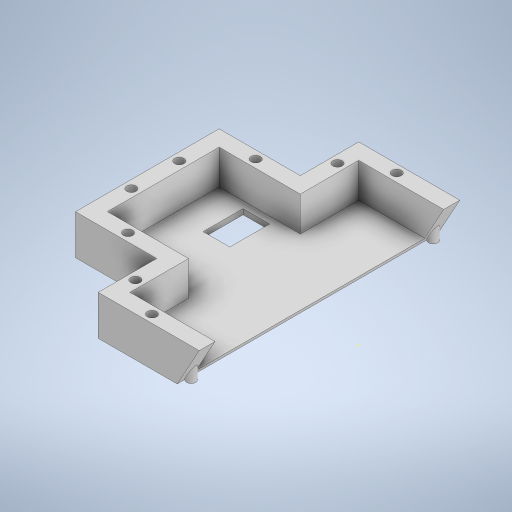
# Autodesk Inventor part: top
Saved by Autodesk Inventor 2023.5 (Build 275446000, 446)
## iProperties
Created: 2025-06-26
Part Number: top
Material: Ogólny
Document SubType Name: Modeling
Designer: karol
Density: 1 g/cm^3
Appearance: Domyślna
Author: karol
Autodesk Inventor part; units mm, degrees
ref_plane "YZ Plane" through (0, 0, 0) normal (1, 0, 0) x (0, 1, 0)
ref_plane "XZ Plane" through (0, 0, 0) normal (0, 1, 0) x (-1, 0, 0)
ref_plane "XY Plane" through (0, 0, 0) normal (0, 0, 1) x (1, 0, 0)
sketch "Szkic1" plane through (0, 0, 0) normal (0, 1, 0) x (-1, 0, 0)
  line L0 (51.2105, 46.6031) -> (4.7105, 46.6031)
  line L1 (4.7105, 46.6031) -> (4.7105, -51.3969)
  line L2 (4.7105, -51.3969) -> (51.2105, -51.3969)
  line L3 (51.2105, -51.3969) -> (51.2105, 46.6031)
  line L4 (51.2105, 46.6031) -> (51.2105, 24.6031)
  line L5 (51.2105, 24.6031) -> (81.7295, 24.6031)
  line L6 (81.7295, 24.6031) -> (81.7295, -29.3969)
  line L7 (81.7295, -29.3969) -> (51.2105, -29.3969)
  line L8 (51.2105, -51.3969) -> (51.2105, -29.3969)
  point P0 (0, 0)
  dimension "d0" = 46.5
  dimension "d1" = 98
  dimension "d2" = 22
  dimension "d3" = 30.519
  dimension "d4" = 54
  constraints: 18 end point, 4 perpendicular, 2 parallel, 2 point on line, 1 collinear, 1 horizontal
  measures "d0" distance of L2.end L1.end
  measures "d1" distance of L1.end L0.end
  measures "d2" distance of L0.start L4.end
  measures "d3" distance of L4.end L5.end
  measures "d4" distance of L5.end L6.end
extrude "Wyciągnięcie proste1" add sketch "Szkic1" along normal blind 15
sketch "Szkic2" plane through (0, 15, 0) normal (0, 1, 0) x (1, 0, 0)
  line L0 (-75.7295, -18.6031) -> (-45.2105, -18.6031)
  line L1 (-45.2105, -18.6031) -> (-45.2105, 23.3969)
  line L2 (-45.2105, 23.3969) -> (-75.7295, 23.3969)
  line L3 (-75.7295, 23.3969) -> (-75.7295, -18.6031)
  line L4 (-81.7295, 29.3969) -> (-81.7295, -24.6031) projected
  line L5 (-81.7295, -24.6031) -> (-51.2105, -24.6031) projected
  line L6 (-45.2105, -40.6509) -> (-10.7105, -40.6509)
  line L7 (-10.7105, -40.6509) -> (-10.7105, 45.3491)
  line L8 (-10.7105, 45.3491) -> (-45.2105, 45.3491)
  line L9 (-45.2105, 45.3491) -> (-45.2105, -40.6509)
  point P0 (0, 0)
  point P1 (-75.7295, 2.3969)
  dimension "d7" = 30.519
  dimension "d8" = 42
  dimension "d9" = 6
  dimension "d10" = 6
  dimension "d11" = 34.5
  dimension "d12" = 86
  constraints: 16 end point, 4 parallel, 2 horizontal, 2 perpendicular, 1 midpoint, 1 point on line
  measures "d7" distance of L2.end L1.end
  measures "d8" distance of L1.end L0.end
  measures "d9" distance from line of L4 point (-75.73, 2.397)
  measures "d10" distance between parallel lines of L5 L0
  measures "d11" distance of L8.end L7.end
  measures "d12" distance of L7.end L6.end
extrude "Wyciągnięcie proste2" cut sketch "Szkic2" against normal blind 13
sketch "Szkic3" plane through (0, 0, 0) normal (0, -1, 0) x (1, 0, 0)
  point P0 (0, 0)
sketch "Szkic4" plane through (0, 0, 0) normal (0, -1, 0) x (1, 0, 0)
  line L0 (-72.6513, -24.862) -> (-72.6513, 21.7196) construction
  line L1 (-72.6513, 21.7196) -> (-57.2809, 21.7196) construction
  line L2 (-57.2809, 21.7196) -> (-57.2809, -24.862) construction
  line L3 (-57.2809, -24.862) -> (-72.6513, -24.862) construction
  line L4 (-66.4228, -19.0142) -> (-66.4228, -19.8248)
  line L5 (-66.4228, -19.8248) -> (-71.6775, -19.8248)
  line L6 (-71.6775, -19.8248) -> (-68.1035, -21.4166)
  line L7 (-68.1035, -21.4166) -> (-68.1035, -21.9109)
  line L8 (-68.1035, -21.9109) -> (-71.6775, -23.4878)
  line L9 (-71.6775, -23.4878) -> (-66.4228, -23.4878)
  line L10 (-66.4228, -23.4878) -> (-66.4228, -24.2441)
  line L11 (-66.4228, -24.2441) -> (-72.5228, -24.2441)
  line L12 (-72.5228, -24.2441) -> (-72.5228, -23.1368)
  line L13 (-72.5228, -23.1368) -> (-69.1267, -21.6143)
  line L14 (-69.1267, -21.6143) -> (-72.5228, -20.1412)
  line L15 (-72.5228, -20.1412) -> (-72.5228, -19.0142)
  line L16 (-72.5228, -19.0142) -> (-66.4228, -19.0142)
  line L17 (-66.4228, -15.6527) -> (-66.4228, -18.0156)
  line L18 (-66.4228, -18.0156) -> (-67.0456, -18.0156)
  line L19 (-67.0456, -18.0156) -> (-67.0456, -17.2395)
  line L20 (-67.0456, -17.2395) -> (-71.8999, -17.2395)
  line L21 (-71.8999, -17.2395) -> (-71.8999, -18.0156)
  line L22 (-71.8999, -18.0156) -> (-72.5228, -18.0156)
  line L23 (-72.5228, -18.0156) -> (-72.5228, -15.6527)
  line L24 (-72.5228, -15.6527) -> (-71.8999, -15.6527)
  line L25 (-71.8999, -15.6527) -> (-71.8999, -16.4288)
  line L26 (-71.8999, -16.4288) -> (-67.0456, -16.4288)
  line L27 (-67.0456, -16.4288) -> (-67.0456, -15.6527)
  line L28 (-67.0456, -15.6527) -> (-66.4228, -15.6527)
  line L29 (-66.4228, -10.2843) -> (-66.4228, -11.1939)
  line L30 (-66.4228, -11.1939) -> (-71.6824, -13.8929)
  line L31 (-71.6824, -13.8929) -> (-66.4228, -13.8929)
  line L32 (-66.4228, -13.8929) -> (-66.4228, -14.6492)
  line L33 (-66.4228, -14.6492) -> (-72.5228, -14.6492)
  line L34 (-72.5228, -14.6492) -> (-72.5228, -13.4975)
  line L35 (-72.5228, -13.4975) -> (-67.6932, -11.0407)
  line L36 (-67.6932, -11.0407) -> (-72.5228, -11.0407)
  line L37 (-72.5228, -11.0407) -> (-72.5228, -10.2843)
  line L38 (-72.5228, -10.2843) -> (-66.4228, -10.2843)
  line L39 (-66.4228, -6.9229) -> (-66.4228, -9.2858)
  line L40 (-66.4228, -9.2858) -> (-67.0456, -9.2858)
  line L41 (-67.0456, -9.2858) -> (-67.0456, -8.5097)
  line L42 (-67.0456, -8.5097) -> (-71.8999, -8.5097)
  line L43 (-71.8999, -8.5097) -> (-71.8999, -9.2858)
  line L44 (-71.8999, -9.2858) -> (-72.5228, -9.2858)
  line L45 (-72.5228, -9.2858) -> (-72.5228, -6.9229)
  line L46 (-72.5228, -6.9229) -> (-71.8999, -6.9229)
  line L47 (-71.8999, -6.9229) -> (-71.8999, -7.699)
  line L48 (-71.8999, -7.699) -> (-67.0456, -7.699)
  line L49 (-67.0456, -7.699) -> (-67.0456, -6.9229)
  line L50 (-67.0456, -6.9229) -> (-66.4228, -6.9229)
  spline S0 degree 2 poles (-68.2963, -1.7819) (-67.8415, -1.7819) (-67.1445, -2.1279) (-66.9171, -2.4146) knots 0 0 0 1 2 2 2
  spline S1 degree 2 poles (-66.9171, -2.4146) (-66.6502, -2.7607) (-66.4228, -3.5466) (-66.4228, -4.1695) knots 0 0 0 1 2 2 2
  line L51 (-66.4228, -4.1695) -> (-66.4228, -5.9194)
  line L52 (-66.4228, -5.9194) -> (-72.5228, -5.9194)
  line L53 (-72.5228, -5.9194) -> (-72.5228, -4.303)
  spline S2 degree 2 poles (-72.5228, -4.303) (-72.5228, -3.6505) (-72.4387, -2.9979) (-72.2756, -2.7013) knots 0 0 0 1 2 2 2
  spline S3 degree 2 poles (-72.2756, -2.7013) (-72.1026, -2.3701) (-71.5341, -2.0686) (-71.1485, -2.0686) knots 0 0 0 1 2 2 2
  spline S4 degree 2 poles (-71.1485, -2.0686) (-70.7185, -2.0686) (-70.0363, -2.5234) (-69.8435, -2.9238) knots 0 0 0 1 2 2 2
  line L54 (-69.8435, -2.9238) -> (-69.8139, -2.9238)
  spline S5 degree 2 poles (-69.8139, -2.9238) (-69.6656, -2.38) (-68.8796, -1.7819) (-68.2963, -1.7819) knots 0 0 0 1 2 2 2
  spline S6 degree 2 poles (-68.2617, -2.6272) (-68.6077, -2.6272) (-69.0526, -2.8249) (-69.2108, -3.1215) knots 0 0 0 1 2 2 2
  spline S7 degree 2 poles (-69.2108, -3.1215) (-69.3096, -3.3143) (-69.369, -3.7691) (-69.369, -4.1893) knots 0 0 0 1 2 2 2
  line L55 (-69.369, -4.1893) -> (-69.369, -5.1087)
  line L56 (-69.369, -5.1087) -> (-67.1148, -5.1087)
  line L57 (-67.1148, -5.1087) -> (-67.1148, -4.4513)
  spline S8 degree 2 poles (-67.1148, -4.4513) (-67.1148, -3.9174) (-67.2137, -3.3044) (-67.3719, -3.0672) knots 0 0 0 1 2 2 2
  spline S9 degree 2 poles (-67.3719, -3.0672) (-67.535, -2.8398) (-67.9403, -2.6272) (-68.2617, -2.6272) knots 0 0 0 1 2 2 2
  spline S10 degree 2 poles (-71.0348, -2.9139) (-71.2523, -2.9139) (-71.5786, -3.0622) (-71.6725, -3.2253) knots 0 0 0 1 2 2 2
  spline S11 degree 2 poles (-71.6725, -3.2253) (-71.7813, -3.4231) (-71.8307, -3.9026) (-71.8307, -4.3326) knots 0 0 0 1 2 2 2
  line L58 (-71.8307, -4.3326) -> (-71.8307, -5.1087)
  line L59 (-71.8307, -5.1087) -> (-70.0462, -5.1087)
  line L60 (-70.0462, -5.1087) -> (-70.0462, -4.1893)
  spline S12 degree 2 poles (-70.0462, -4.1893) (-70.0462, -3.8086) (-70.1253, -3.4478) (-70.2489, -3.255) knots 0 0 0 1 2 2 2
  spline S13 degree 2 poles (-70.2489, -3.255) (-70.3675, -3.0672) (-70.7481, -2.9139) (-71.0348, -2.9139) knots 0 0 0 1 2 2 2
  spline S14 degree 2 poles (-71.8258, 3.3393) (-71.4204, 3.6854) (-70.234, 4.0709) (-69.4728, 4.0709) knots 0 0 0 1 2 2 2
  spline S15 degree 2 poles (-69.4728, 4.0709) (-68.7313, 4.0709) (-67.5301, 3.6952) (-67.1247, 3.3393) knots 0 0 0 1 2 2 2
  spline S16 degree 2 poles (-67.1247, 3.3393) (-66.6996, 2.9636) (-66.2942, 1.97) (-66.2942, 1.3719) knots 0 0 0 1 2 2 2
  spline S17 degree 2 poles (-66.2942, 1.3719) (-66.2942, 0.754) (-66.7144, -0.2347) (-67.1247, -0.5955) knots 0 0 0 1 2 2 2
  spline S18 degree 2 poles (-67.1247, -0.5955) (-67.5301, -0.9465) (-68.7214, -1.3222) (-69.4728, -1.3222) knots 0 0 0 1 2 2 2
  spline S19 degree 2 poles (-69.4728, -1.3222) (-70.239, -1.3222) (-71.4056, -0.9415) (-71.8258, -0.5906) knots 0 0 0 1 2 2 2
  spline S20 degree 2 poles (-71.8258, -0.5906) (-72.2311, -0.2347) (-72.6513, 0.7589) (-72.6513, 1.3719) knots 0 0 0 1 2 2 2
  spline S21 degree 2 poles (-72.6513, 1.3719) (-72.6513, 1.9948) (-72.2163, 2.9933) (-71.8258, 3.3393) knots 0 0 0 1 2 2 2
  spline S22 degree 2 poles (-69.4728, 3.2256) (-70.0758, 3.2256) (-71.0101, 2.9636) (-71.3166, 2.7264) knots 0 0 0 1 2 2 2
  spline S23 degree 2 poles (-71.3166, 2.7264) (-71.633, 2.4841) (-71.9493, 1.802) (-71.9493, 1.3769) knots 0 0 0 1 2 2 2
  spline S24 degree 2 poles (-71.9493, 1.3769) (-71.9493, 0.9369) (-71.6429, 0.2745) (-71.3166, 0.0224) knots 0 0 0 1 2 2 2
  spline S25 degree 2 poles (-71.3166, 0.0224) (-71.0052, -0.2198) (-70.066, -0.4769) (-69.4728, -0.4769) knots 0 0 0 1 2 2 2
  spline S26 degree 2 poles (-69.4728, -0.4769) (-68.2715, -0.4769) (-66.9962, 0.5316) (-66.9962, 1.3769) knots 0 0 0 1 2 2 2
  spline S27 degree 2 poles (-66.9962, 1.3769) (-66.9962, 2.2222) (-68.2715, 3.2256) (-69.4728, 3.2256) knots 0 0 0 1 2 2 2
  line L61 (-66.4228, 8.4952) -> (-66.4228, 4.9607)
  line L62 (-66.4228, 4.9607) -> (-72.5228, 4.9607)
  line L63 (-72.5228, 4.9607) -> (-72.5228, 5.7714)
  line L64 (-72.5228, 5.7714) -> (-67.1445, 5.7714)
  line L65 (-67.1445, 5.7714) -> (-67.1445, 8.4952)
  line L66 (-67.1445, 8.4952) -> (-66.4228, 8.4952)
  line L67 (-66.4228, 10.5565) -> (-71.801, 10.5565)
  line L68 (-71.801, 10.5565) -> (-71.801, 8.51)
  line L69 (-71.801, 8.51) -> (-72.5228, 8.51)
  line L70 (-72.5228, 8.51) -> (-72.5228, 13.4137)
  line L71 (-72.5228, 13.4137) -> (-71.801, 13.4137)
  line L72 (-71.801, 13.4137) -> (-71.801, 11.3672)
  line L73 (-71.801, 11.3672) -> (-66.4228, 11.3672)
  line L74 (-66.4228, 11.3672) -> (-66.4228, 10.5565)
  line L75 (-60.0728, 0.0946) -> (-60.0728, -0.8738)
  line L76 (-60.0728, -0.8738) -> (-61.2365, -1.755)
  line L77 (-61.2365, -1.755) -> (-61.2365, -2.0427)
  line L78 (-61.2365, -2.0427) -> (-60.0728, -2.0427)
  line L79 (-60.0728, -2.0427) -> (-60.0728, -2.8339)
  line L80 (-60.0728, -2.8339) -> (-63.2428, -2.8339)
  line L81 (-63.2428, -2.8339) -> (-63.2428, -1.5597)
  spline S28 degree 2 poles (-63.2428, -1.5597) (-63.2428, -1.2951) (-63.176, -0.9047) (-63.0732, -0.7377) knots 0 0 0 1 2 2 2
  spline S29 degree 2 poles (-63.0732, -0.7377) (-62.9653, -0.5681) (-62.6288, -0.3678) (-62.3719, -0.3678) knots 0 0 0 1 2 2 2
  spline S30 degree 2 poles (-62.3719, -0.3678) (-62.0097, -0.3678) (-61.555, -0.6966) (-61.4214, -0.9714) knots 0 0 0 1 2 2 2
  line L82 (-61.4214, -0.9714) -> (-60.0728, 0.0946)
  spline S31 degree 2 poles (-62.2717, -1.1847) (-62.3925, -1.1847) (-62.5646, -1.2771) (-62.6108, -1.3825) knots 0 0 0 1 2 2 2
  spline S32 degree 2 poles (-62.6108, -1.3825) (-62.6417, -1.457) (-62.6596, -1.6394) (-62.6596, -1.7755) knots 0 0 0 1 2 2 2
  line L83 (-62.6596, -1.7755) -> (-62.6596, -2.0427)
  line L84 (-62.6596, -2.0427) -> (-61.8068, -2.0427)
  line L85 (-61.8068, -2.0427) -> (-61.8068, -1.814)
  spline S33 degree 2 poles (-61.8068, -1.814) (-61.8068, -1.6496) (-61.8479, -1.4159) (-61.9121, -1.3362) knots 0 0 0 1 2 2 2
  spline S34 degree 2 poles (-61.9121, -1.3362) (-61.9737, -1.2592) (-62.1382, -1.1847) (-62.2717, -1.1847) knots 0 0 0 1 2 2 2
  spline S35 degree 2 poles (-61.6578, 3.2158) (-60.8871, 3.2158) (-60.006, 2.3938) (-60.006, 1.6796) knots 0 0 0 1 2 2 2
  spline S36 degree 2 poles (-60.006, 1.6796) (-60.006, 0.9629) (-60.8974, 0.146) (-61.6578, 0.146) knots 0 0 0 1 2 2 2
  spline S37 degree 2 poles (-61.6578, 0.146) (-62.4207, 0.146) (-63.3096, 0.9629) (-63.3096, 1.6796) knots 0 0 0 1 2 2 2
  spline S38 degree 2 poles (-63.3096, 1.6796) (-63.3096, 2.3938) (-62.4259, 3.2158) (-61.6578, 3.2158) knots 0 0 0 1 2 2 2
  spline S39 degree 2 poles (-61.6578, 2.3938) (-61.9429, 2.3938) (-62.3411, 2.2782) (-62.467, 2.178) knots 0 0 0 1 2 2 2
  spline S40 degree 2 poles (-62.467, 2.178) (-62.598, 2.0778) (-62.711, 1.8209) (-62.711, 1.6822) knots 0 0 0 1 2 2 2
  spline S41 degree 2 poles (-62.711, 1.6822) (-62.711, 1.5358) (-62.6057, 1.2969) (-62.4721, 1.1864) knots 0 0 0 1 2 2 2
  spline S42 degree 2 poles (-62.4721, 1.1864) (-62.3488, 1.0888) (-61.9403, 0.9681) (-61.6578, 0.9681) knots 0 0 0 1 2 2 2
  spline S43 degree 2 poles (-61.6578, 0.9681) (-61.3649, 0.9681) (-60.9796, 1.0837) (-60.8486, 1.1838) knots 0 0 0 1 2 2 2
  spline S44 degree 2 poles (-60.8486, 1.1838) (-60.7176, 1.284) (-60.6045, 1.5435) (-60.6045, 1.6822) knots 0 0 0 1 2 2 2
  spline S45 degree 2 poles (-60.6045, 1.6822) (-60.6045, 1.8235) (-60.7253, 2.0855) (-60.8537, 2.1806) knots 0 0 0 1 2 2 2
  spline S46 degree 2 poles (-60.8537, 2.1806) (-60.9924, 2.2833) (-61.3598, 2.3938) (-61.6578, 2.3938) knots 0 0 0 1 2 2 2
  spline S47 degree 2 poles (-61.0438, 6.2214) (-60.8075, 6.2214) (-60.4504, 6.0416) (-60.3322, 5.8926) knots 0 0 0 1 2 2 2
  spline S48 degree 2 poles (-60.3322, 5.8926) (-60.1909, 5.7128) (-60.0728, 5.2863) (-60.0728, 4.955) knots 0 0 0 1 2 2 2
  line L86 (-60.0728, 4.955) -> (-60.0728, 3.6885)
  line L87 (-60.0728, 3.6885) -> (-63.2428, 3.6885)
  line L88 (-63.2428, 3.6885) -> (-63.2428, 4.806)
  spline S49 degree 2 poles (-63.2428, 4.806) (-63.2428, 5.1553) (-63.1888, 5.515) (-63.1041, 5.6717) knots 0 0 0 1 2 2 2
  spline S50 degree 2 poles (-63.1041, 5.6717) (-63.0141, 5.8438) (-62.7059, 6.0108) (-62.5055, 6.0108) knots 0 0 0 1 2 2 2
  spline S51 degree 2 poles (-62.5055, 6.0108) (-62.2743, 6.0108) (-61.9121, 5.7796) (-61.8273, 5.5741) knots 0 0 0 1 2 2 2
  line L89 (-61.8273, 5.5741) -> (-61.8119, 5.5741)
  spline S52 degree 2 poles (-61.8119, 5.5741) (-61.7503, 5.8695) (-61.3675, 6.2214) (-61.0438, 6.2214) knots 0 0 0 1 2 2 2
  spline S53 degree 2 poles (-61.0567, 5.3994) (-61.2056, 5.3994) (-61.3726, 5.2812) (-61.4163, 5.163) knots 0 0 0 1 2 2 2
  spline S54 degree 2 poles (-61.4163, 5.163) (-61.4446, 5.0911) (-61.4497, 4.8368) (-61.4497, 4.6261) knots 0 0 0 1 2 2 2
  line L90 (-61.4497, 4.6261) -> (-61.4497, 4.4797)
  line L91 (-61.4497, 4.4797) -> (-60.6508, 4.4797)
  line L92 (-60.6508, 4.4797) -> (-60.6508, 4.5234)
  spline S55 degree 2 poles (-60.6508, 4.5234) (-60.6508, 4.8317) (-60.6585, 5.068) (-60.7124, 5.1913) knots 0 0 0 1 2 2 2
  spline S56 degree 2 poles (-60.7124, 5.1913) (-60.7612, 5.2992) (-60.9411, 5.3994) (-61.0567, 5.3994) knots 0 0 0 1 2 2 2
  spline S57 degree 2 poles (-62.3488, 5.2016) (-62.4259, 5.2016) (-62.5877, 5.1219) (-62.6237, 5.0397) knots 0 0 0 1 2 2 2
  spline S58 degree 2 poles (-62.6237, 5.0397) (-62.6596, 4.9627) (-62.6648, 4.7469) (-62.6648, 4.5337) knots 0 0 0 1 2 2 2
  line L93 (-62.6648, 4.5337) -> (-62.6648, 4.4797)
  line L94 (-62.6648, 4.4797) -> (-61.9917, 4.4797)
  line L95 (-61.9917, 4.4797) -> (-61.9917, 4.5799)
  spline S59 degree 2 poles (-61.9917, 4.5799) (-61.9917, 4.7828) (-61.9994, 4.9473) (-62.0405, 5.0346) knots 0 0 0 1 2 2 2
  spline S60 degree 2 poles (-62.0405, 5.0346) (-62.0868, 5.1296) (-62.2435, 5.2016) (-62.3488, 5.2016) knots 0 0 0 1 2 2 2
  spline S61 degree 2 poles (-61.6578, 9.5635) (-60.8871, 9.5635) (-60.006, 8.7415) (-60.006, 8.0273) knots 0 0 0 1 2 2 2
  spline S62 degree 2 poles (-60.006, 8.0273) (-60.006, 7.3106) (-60.8974, 6.4937) (-61.6578, 6.4937) knots 0 0 0 1 2 2 2
  spline S63 degree 2 poles (-61.6578, 6.4937) (-62.4207, 6.4937) (-63.3096, 7.3106) (-63.3096, 8.0273) knots 0 0 0 1 2 2 2
  spline S64 degree 2 poles (-63.3096, 8.0273) (-63.3096, 8.7415) (-62.4259, 9.5635) (-61.6578, 9.5635) knots 0 0 0 1 2 2 2
  spline S65 degree 2 poles (-61.6578, 8.7415) (-61.9429, 8.7415) (-62.3411, 8.6259) (-62.467, 8.5257) knots 0 0 0 1 2 2 2
  spline S66 degree 2 poles (-62.467, 8.5257) (-62.598, 8.4255) (-62.711, 8.1686) (-62.711, 8.0299) knots 0 0 0 1 2 2 2
  spline S67 degree 2 poles (-62.711, 8.0299) (-62.711, 7.8835) (-62.6057, 7.6446) (-62.4721, 7.5341) knots 0 0 0 1 2 2 2
  spline S68 degree 2 poles (-62.4721, 7.5341) (-62.3488, 7.4365) (-61.9403, 7.3158) (-61.6578, 7.3158) knots 0 0 0 1 2 2 2
  spline S69 degree 2 poles (-61.6578, 7.3158) (-61.3649, 7.3158) (-60.9796, 7.4314) (-60.8486, 7.5316) knots 0 0 0 1 2 2 2
  spline S70 degree 2 poles (-60.8486, 7.5316) (-60.7176, 7.6317) (-60.6045, 7.8912) (-60.6045, 8.0299) knots 0 0 0 1 2 2 2
  spline S71 degree 2 poles (-60.6045, 8.0299) (-60.6045, 8.1712) (-60.7253, 8.4332) (-60.8537, 8.5283) knots 0 0 0 1 2 2 2
  spline S72 degree 2 poles (-60.8537, 8.5283) (-60.9924, 8.631) (-61.3598, 8.7415) (-61.6578, 8.7415) knots 0 0 0 1 2 2 2
  line L96 (-60.0728, 11.6135) -> (-60.0728, 9.9078)
  line L97 (-60.0728, 9.9078) -> (-60.6251, 9.9078)
  line L98 (-60.6251, 9.9078) -> (-60.6251, 10.3625)
  line L99 (-60.6251, 10.3625) -> (-62.6905, 10.3625)
  line L100 (-62.6905, 10.3625) -> (-62.6905, 9.9078)
  line L101 (-62.6905, 9.9078) -> (-63.2428, 9.9078)
  line L102 (-63.2428, 9.9078) -> (-63.2428, 11.6135)
  line L103 (-63.2428, 11.6135) -> (-62.6905, 11.6135)
  line L104 (-62.6905, 11.6135) -> (-62.6905, 11.1588)
  line L105 (-62.6905, 11.1588) -> (-60.6251, 11.1588)
  line L106 (-60.6251, 11.1588) -> (-60.6251, 11.6135)
  line L107 (-60.6251, 11.6135) -> (-60.0728, 11.6135)
  line L108 (-60.0728, 14.2569) -> (-60.0728, 12.1427)
  line L109 (-60.0728, 12.1427) -> (-63.2428, 12.1427)
  line L110 (-63.2428, 12.1427) -> (-63.2428, 12.939)
  line L111 (-63.2428, 12.939) -> (-60.6765, 12.939)
  line L112 (-60.6765, 12.939) -> (-60.6765, 14.2569)
  line L113 (-60.6765, 14.2569) -> (-60.0728, 14.2569)
  spline S73 degree 2 poles (-61.6578, 17.5219) (-60.8871, 17.5219) (-60.006, 16.6999) (-60.006, 15.9857) knots 0 0 0 1 2 2 2
  spline S74 degree 2 poles (-60.006, 15.9857) (-60.006, 15.269) (-60.8974, 14.4521) (-61.6578, 14.4521) knots 0 0 0 1 2 2 2
  spline S75 degree 2 poles (-61.6578, 14.4521) (-62.4207, 14.4521) (-63.3096, 15.269) (-63.3096, 15.9857) knots 0 0 0 1 2 2 2
  spline S76 degree 2 poles (-63.3096, 15.9857) (-63.3096, 16.6999) (-62.4259, 17.5219) (-61.6578, 17.5219) knots 0 0 0 1 2 2 2
  spline S77 degree 2 poles (-61.6578, 16.6999) (-61.9429, 16.6999) (-62.3411, 16.5843) (-62.467, 16.4841) knots 0 0 0 1 2 2 2
  spline S78 degree 2 poles (-62.467, 16.4841) (-62.598, 16.3839) (-62.711, 16.127) (-62.711, 15.9883) knots 0 0 0 1 2 2 2
  spline S79 degree 2 poles (-62.711, 15.9883) (-62.711, 15.8419) (-62.6057, 15.603) (-62.4721, 15.4925) knots 0 0 0 1 2 2 2
  spline S80 degree 2 poles (-62.4721, 15.4925) (-62.3488, 15.3949) (-61.9403, 15.2742) (-61.6578, 15.2742) knots 0 0 0 1 2 2 2
  spline S81 degree 2 poles (-61.6578, 15.2742) (-61.3649, 15.2742) (-60.9796, 15.3898) (-60.8486, 15.4899) knots 0 0 0 1 2 2 2
  spline S82 degree 2 poles (-60.8486, 15.4899) (-60.7176, 15.5901) (-60.6045, 15.8496) (-60.6045, 15.9883) knots 0 0 0 1 2 2 2
  spline S83 degree 2 poles (-60.6045, 15.9883) (-60.6045, 16.1296) (-60.7253, 16.3916) (-60.8537, 16.4867) knots 0 0 0 1 2 2 2
  spline S84 degree 2 poles (-60.8537, 16.4867) (-60.9924, 16.5894) (-61.3598, 16.6999) (-61.6578, 16.6999) knots 0 0 0 1 2 2 2
  point P0 (0, 0)
  constraints: 2 other
extrude "Wyciągnięcie proste3" add sketch "Szkic4" against normal blind 1
sketch "Szkic5" plane through (0, 0, 0) normal (0, -1, 0) x (1, 0, 0)
  point P0 (0, 0)
sketch "Szkic6" plane through (0, 0, 0) normal (0, -1, 0) x (1, 0, 0)
  line L0 (-74.9036, -23.2743) -> (-74.9036, 27.821) construction
  line L1 (-74.9036, 27.821) -> (-59.7073, 27.821) construction
  line L2 (-59.7073, 27.821) -> (-59.7073, -23.2743) construction
  line L3 (-59.7073, -23.2743) -> (-74.9036, -23.2743) construction
  line L4 (-68.6751, -17.4264) -> (-68.6751, -18.2371)
  line L5 (-68.6751, -18.2371) -> (-73.9298, -18.2371)
  line L6 (-73.9298, -18.2371) -> (-70.3558, -19.8289)
  line L7 (-70.3558, -19.8289) -> (-70.3558, -20.3232)
  line L8 (-70.3558, -20.3232) -> (-73.9298, -21.9001)
  line L9 (-73.9298, -21.9001) -> (-68.6751, -21.9001)
  line L10 (-68.6751, -21.9001) -> (-68.6751, -22.6564)
  line L11 (-68.6751, -22.6564) -> (-74.7751, -22.6564)
  line L12 (-74.7751, -22.6564) -> (-74.7751, -21.5491)
  line L13 (-74.7751, -21.5491) -> (-71.379, -20.0266)
  line L14 (-71.379, -20.0266) -> (-74.7751, -18.5535)
  line L15 (-74.7751, -18.5535) -> (-74.7751, -17.4264)
  line L16 (-74.7751, -17.4264) -> (-68.6751, -17.4264)
  line L17 (-68.6751, -14.065) -> (-68.6751, -16.4279)
  line L18 (-68.6751, -16.4279) -> (-69.2979, -16.4279)
  line L19 (-69.2979, -16.4279) -> (-69.2979, -15.6518)
  line L20 (-69.2979, -15.6518) -> (-74.1522, -15.6518)
  line L21 (-74.1522, -15.6518) -> (-74.1522, -16.4279)
  line L22 (-74.1522, -16.4279) -> (-74.7751, -16.4279)
  line L23 (-74.7751, -16.4279) -> (-74.7751, -14.065)
  line L24 (-74.7751, -14.065) -> (-74.1522, -14.065)
  line L25 (-74.1522, -14.065) -> (-74.1522, -14.8411)
  line L26 (-74.1522, -14.8411) -> (-69.2979, -14.8411)
  line L27 (-69.2979, -14.8411) -> (-69.2979, -14.065)
  line L28 (-69.2979, -14.065) -> (-68.6751, -14.065)
  line L29 (-68.6751, -8.6966) -> (-68.6751, -9.6062)
  line L30 (-68.6751, -9.6062) -> (-73.9347, -12.3052)
  line L31 (-73.9347, -12.3052) -> (-68.6751, -12.3052)
  line L32 (-68.6751, -12.3052) -> (-68.6751, -13.0615)
  line L33 (-68.6751, -13.0615) -> (-74.7751, -13.0615)
  line L34 (-74.7751, -13.0615) -> (-74.7751, -11.9097)
  line L35 (-74.7751, -11.9097) -> (-69.9455, -9.4529)
  line L36 (-69.9455, -9.4529) -> (-74.7751, -9.4529)
  line L37 (-74.7751, -9.4529) -> (-74.7751, -8.6966)
  line L38 (-74.7751, -8.6966) -> (-68.6751, -8.6966)
  line L39 (-68.6751, -5.3352) -> (-68.6751, -7.6981)
  line L40 (-68.6751, -7.6981) -> (-69.2979, -7.6981)
  line L41 (-69.2979, -7.6981) -> (-69.2979, -6.922)
  line L42 (-69.2979, -6.922) -> (-74.1522, -6.922)
  line L43 (-74.1522, -6.922) -> (-74.1522, -7.6981)
  line L44 (-74.1522, -7.6981) -> (-74.7751, -7.6981)
  line L45 (-74.7751, -7.6981) -> (-74.7751, -5.3352)
  line L46 (-74.7751, -5.3352) -> (-74.1522, -5.3352)
  line L47 (-74.1522, -5.3352) -> (-74.1522, -6.1113)
  line L48 (-74.1522, -6.1113) -> (-69.2979, -6.1113)
  line L49 (-69.2979, -6.1113) -> (-69.2979, -5.3352)
  line L50 (-69.2979, -5.3352) -> (-68.6751, -5.3352)
  spline S0 degree 2 poles (-70.5486, -0.1942) (-70.0938, -0.1942) (-69.3968, -0.5402) (-69.1694, -0.8269) knots 0 0 0 1 2 2 2
  spline S1 degree 2 poles (-69.1694, -0.8269) (-68.9025, -1.1729) (-68.6751, -1.9589) (-68.6751, -2.5818) knots 0 0 0 1 2 2 2
  line L51 (-68.6751, -2.5818) -> (-68.6751, -4.3317)
  line L52 (-68.6751, -4.3317) -> (-74.7751, -4.3317)
  line L53 (-74.7751, -4.3317) -> (-74.7751, -2.7152)
  spline S2 degree 2 poles (-74.7751, -2.7152) (-74.7751, -2.0627) (-74.691, -1.4102) (-74.5279, -1.1136) knots 0 0 0 1 2 2 2
  spline S3 degree 2 poles (-74.5279, -1.1136) (-74.3549, -0.7824) (-73.7864, -0.4809) (-73.4008, -0.4809) knots 0 0 0 1 2 2 2
  spline S4 degree 2 poles (-73.4008, -0.4809) (-72.9708, -0.4809) (-72.2886, -0.9357) (-72.0958, -1.3361) knots 0 0 0 1 2 2 2
  line L54 (-72.0958, -1.3361) -> (-72.0662, -1.3361)
  spline S5 degree 2 poles (-72.0662, -1.3361) (-71.9179, -0.7923) (-71.1319, -0.1942) (-70.5486, -0.1942) knots 0 0 0 1 2 2 2
  spline S6 degree 2 poles (-70.514, -1.0395) (-70.86, -1.0395) (-71.3049, -1.2372) (-71.4631, -1.5338) knots 0 0 0 1 2 2 2
  spline S7 degree 2 poles (-71.4631, -1.5338) (-71.5619, -1.7266) (-71.6213, -2.1814) (-71.6213, -2.6016) knots 0 0 0 1 2 2 2
  line L55 (-71.6213, -2.6016) -> (-71.6213, -3.521)
  line L56 (-71.6213, -3.521) -> (-69.3671, -3.521)
  line L57 (-69.3671, -3.521) -> (-69.3671, -2.8635)
  spline S8 degree 2 poles (-69.3671, -2.8635) (-69.3671, -2.3297) (-69.466, -1.7167) (-69.6242, -1.4794) knots 0 0 0 1 2 2 2
  spline S9 degree 2 poles (-69.6242, -1.4794) (-69.7873, -1.252) (-70.1927, -1.0395) (-70.514, -1.0395) knots 0 0 0 1 2 2 2
  spline S10 degree 2 poles (-73.2871, -1.3262) (-73.5046, -1.3262) (-73.8309, -1.4745) (-73.9248, -1.6376) knots 0 0 0 1 2 2 2
  spline S11 degree 2 poles (-73.9248, -1.6376) (-74.0336, -1.8353) (-74.083, -2.3148) (-74.083, -2.7449) knots 0 0 0 1 2 2 2
  line L58 (-74.083, -2.7449) -> (-74.083, -3.521)
  line L59 (-74.083, -3.521) -> (-72.2985, -3.521)
  line L60 (-72.2985, -3.521) -> (-72.2985, -2.6016)
  spline S12 degree 2 poles (-72.2985, -2.6016) (-72.2985, -2.2209) (-72.3776, -1.8601) (-72.5012, -1.6673) knots 0 0 0 1 2 2 2
  spline S13 degree 2 poles (-72.5012, -1.6673) (-72.6198, -1.4794) (-73.0004, -1.3262) (-73.2871, -1.3262) knots 0 0 0 1 2 2 2
  spline S14 degree 2 poles (-74.0781, 4.9271) (-73.6727, 5.2731) (-72.4863, 5.6587) (-71.7251, 5.6587) knots 0 0 0 1 2 2 2
  spline S15 degree 2 poles (-71.7251, 5.6587) (-70.9836, 5.6587) (-69.7824, 5.283) (-69.377, 4.9271) knots 0 0 0 1 2 2 2
  spline S16 degree 2 poles (-69.377, 4.9271) (-68.9519, 4.5514) (-68.5465, 3.5578) (-68.5465, 2.9596) knots 0 0 0 1 2 2 2
  spline S17 degree 2 poles (-68.5465, 2.9596) (-68.5465, 2.3417) (-68.9667, 1.3531) (-69.377, 0.9922) knots 0 0 0 1 2 2 2
  spline S18 degree 2 poles (-69.377, 0.9922) (-69.7824, 0.6412) (-70.9737, 0.2655) (-71.7251, 0.2655) knots 0 0 0 1 2 2 2
  spline S19 degree 2 poles (-71.7251, 0.2655) (-72.4913, 0.2655) (-73.6579, 0.6462) (-74.0781, 0.9971) knots 0 0 0 1 2 2 2
  spline S20 degree 2 poles (-74.0781, 0.9971) (-74.4834, 1.3531) (-74.9036, 2.3467) (-74.9036, 2.9596) knots 0 0 0 1 2 2 2
  spline S21 degree 2 poles (-74.9036, 2.9596) (-74.9036, 3.5825) (-74.4686, 4.581) (-74.0781, 4.9271) knots 0 0 0 1 2 2 2
  spline S22 degree 2 poles (-71.7251, 4.8134) (-72.3281, 4.8134) (-73.2624, 4.5514) (-73.5689, 4.3141) knots 0 0 0 1 2 2 2
  spline S23 degree 2 poles (-73.5689, 4.3141) (-73.8853, 4.0719) (-74.2016, 3.3897) (-74.2016, 2.9646) knots 0 0 0 1 2 2 2
  spline S24 degree 2 poles (-74.2016, 2.9646) (-74.2016, 2.5246) (-73.8952, 1.8622) (-73.5689, 1.6101) knots 0 0 0 1 2 2 2
  spline S25 degree 2 poles (-73.5689, 1.6101) (-73.2575, 1.3679) (-72.3183, 1.1108) (-71.7251, 1.1108) knots 0 0 0 1 2 2 2
  spline S26 degree 2 poles (-71.7251, 1.1108) (-70.5239, 1.1108) (-69.2485, 2.1193) (-69.2485, 2.9646) knots 0 0 0 1 2 2 2
  spline S27 degree 2 poles (-69.2485, 2.9646) (-69.2485, 3.8099) (-70.5239, 4.8134) (-71.7251, 4.8134) knots 0 0 0 1 2 2 2
  line L61 (-68.6751, 10.0829) -> (-68.6751, 6.5484)
  line L62 (-68.6751, 6.5484) -> (-74.7751, 6.5484)
  line L63 (-74.7751, 6.5484) -> (-74.7751, 7.3591)
  line L64 (-74.7751, 7.3591) -> (-69.3968, 7.3591)
  line L65 (-69.3968, 7.3591) -> (-69.3968, 10.0829)
  line L66 (-69.3968, 10.0829) -> (-68.6751, 10.0829)
  line L67 (-68.6751, 12.1442) -> (-74.0533, 12.1442)
  line L68 (-74.0533, 12.1442) -> (-74.0533, 10.0977)
  line L69 (-74.0533, 10.0977) -> (-74.7751, 10.0977)
  line L70 (-74.7751, 10.0977) -> (-74.7751, 15.0014)
  line L71 (-74.7751, 15.0014) -> (-74.0533, 15.0014)
  line L72 (-74.0533, 15.0014) -> (-74.0533, 12.9549)
  line L73 (-74.0533, 12.9549) -> (-68.6751, 12.9549)
  line L74 (-68.6751, 12.9549) -> (-68.6751, 12.1442)
  line L75 (-62.3251, -0.0773) -> (-62.3251, -0.6245)
  line L76 (-62.3251, -0.6245) -> (-63.5864, -1.6264)
  line L77 (-63.5864, -1.6264) -> (-63.5864, -2.1093)
  line L78 (-63.5864, -2.1093) -> (-62.3251, -2.1093)
  line L79 (-62.3251, -2.1093) -> (-62.3251, -2.5306)
  line L80 (-62.3251, -2.5306) -> (-65.4951, -2.5306)
  line L81 (-65.4951, -2.5306) -> (-65.4951, -1.7137)
  spline S28 degree 2 poles (-65.4951, -1.7137) (-65.4951, -1.4414) (-65.436, -1.0741) (-65.3281, -0.9071) knots 0 0 0 1 2 2 2
  spline S29 degree 2 poles (-65.3281, -0.9071) (-65.2202, -0.7401) (-64.8837, -0.5474) (-64.6345, -0.5474) knots 0 0 0 1 2 2 2
  spline S30 degree 2 poles (-64.6345, -0.5474) (-64.2877, -0.5474) (-63.8176, -0.9019) (-63.7046, -1.2051) knots 0 0 0 1 2 2 2
  line L82 (-63.7046, -1.2051) -> (-62.3251, -0.0773)
  spline S31 degree 2 poles (-64.6011, -0.9867) (-64.7398, -0.9867) (-64.953, -1.0843) (-65.0224, -1.1871) knots 0 0 0 1 2 2 2
  spline S32 degree 2 poles (-65.0224, -1.1871) (-65.0815, -1.277) (-65.1303, -1.5159) (-65.1303, -1.6906) knots 0 0 0 1 2 2 2
  line L83 (-65.1303, -1.6906) -> (-65.1303, -2.1093)
  line L84 (-65.1303, -2.1093) -> (-63.9383, -2.1093)
  line L85 (-63.9383, -2.1093) -> (-63.9383, -1.7394)
  spline S33 degree 2 poles (-63.9383, -1.7394) (-63.9383, -1.557) (-64.0026, -1.2667) (-64.1027, -1.1665) knots 0 0 0 1 2 2 2
  spline S34 degree 2 poles (-64.1027, -1.1665) (-64.1901, -1.0741) (-64.4367, -0.9867) (-64.6011, -0.9867) knots 0 0 0 1 2 2 2
  spline S35 degree 2 poles (-65.1329, 2.4171) (-64.9222, 2.5969) (-64.3057, 2.7973) (-63.9101, 2.7973) knots 0 0 0 1 2 2 2
  spline S36 degree 2 poles (-63.9101, 2.7973) (-63.5247, 2.7973) (-62.9005, 2.602) (-62.6899, 2.4171) knots 0 0 0 1 2 2 2
  spline S37 degree 2 poles (-62.6899, 2.4171) (-62.4689, 2.2218) (-62.2583, 1.7055) (-62.2583, 1.3946) knots 0 0 0 1 2 2 2
  spline S38 degree 2 poles (-62.2583, 1.3946) (-62.2583, 1.0735) (-62.4766, 0.5598) (-62.6899, 0.3722) knots 0 0 0 1 2 2 2
  spline S39 degree 2 poles (-62.6899, 0.3722) (-62.9005, 0.1898) (-63.5196, -0.0054) (-63.9101, -0.0054) knots 0 0 0 1 2 2 2
  spline S40 degree 2 poles (-63.9101, -0.0054) (-64.3083, -0.0054) (-64.9145, 0.1924) (-65.1329, 0.3748) knots 0 0 0 1 2 2 2
  spline S41 degree 2 poles (-65.1329, 0.3748) (-65.3435, 0.5598) (-65.5619, 1.0761) (-65.5619, 1.3946) knots 0 0 0 1 2 2 2
  spline S42 degree 2 poles (-65.5619, 1.3946) (-65.5619, 1.7183) (-65.3358, 2.2372) (-65.1329, 2.4171) knots 0 0 0 1 2 2 2
  spline S43 degree 2 poles (-63.9101, 2.358) (-64.2235, 2.358) (-64.709, 2.2218) (-64.8683, 2.0985) knots 0 0 0 1 2 2 2
  spline S44 degree 2 poles (-64.8683, 2.0985) (-65.0327, 1.9726) (-65.1971, 1.6181) (-65.1971, 1.3972) knots 0 0 0 1 2 2 2
  spline S45 degree 2 poles (-65.1971, 1.3972) (-65.1971, 1.1686) (-65.0378, 0.8244) (-64.8683, 0.6933) knots 0 0 0 1 2 2 2
  spline S46 degree 2 poles (-64.8683, 0.6933) (-64.7064, 0.5675) (-64.2183, 0.4339) (-63.9101, 0.4339) knots 0 0 0 1 2 2 2
  spline S47 degree 2 poles (-63.9101, 0.4339) (-63.2858, 0.4339) (-62.6231, 0.9579) (-62.6231, 1.3972) knots 0 0 0 1 2 2 2
  spline S48 degree 2 poles (-62.6231, 1.3972) (-62.6231, 1.8365) (-63.2858, 2.358) (-63.9101, 2.358) knots 0 0 0 1 2 2 2
  spline S49 degree 2 poles (-63.2987, 5.4098) (-63.0623, 5.4098) (-62.7001, 5.23) (-62.582, 5.081) knots 0 0 0 1 2 2 2
  spline S50 degree 2 poles (-62.582, 5.081) (-62.4432, 4.9012) (-62.3251, 4.4927) (-62.3251, 4.169) knots 0 0 0 1 2 2 2
  line L86 (-62.3251, 4.169) -> (-62.3251, 3.2597)
  line L87 (-62.3251, 3.2597) -> (-65.4951, 3.2597)
  line L88 (-65.4951, 3.2597) -> (-65.4951, 4.0997)
  spline S51 degree 2 poles (-65.4951, 4.0997) (-65.4951, 4.4388) (-65.4514, 4.7779) (-65.3666, 4.932) knots 0 0 0 1 2 2 2
  spline S52 degree 2 poles (-65.3666, 4.932) (-65.2767, 5.1041) (-64.9813, 5.2608) (-64.7809, 5.2608) knots 0 0 0 1 2 2 2
  spline S53 degree 2 poles (-64.7809, 5.2608) (-64.5574, 5.2608) (-64.2029, 5.0245) (-64.1027, 4.8164) knots 0 0 0 1 2 2 2
  line L89 (-64.1027, 4.8164) -> (-64.0873, 4.8164)
  spline S54 degree 2 poles (-64.0873, 4.8164) (-64.0103, 5.099) (-63.6018, 5.4098) (-63.2987, 5.4098) knots 0 0 0 1 2 2 2
  spline S55 degree 2 poles (-63.2807, 4.9705) (-63.4605, 4.9705) (-63.6917, 4.8678) (-63.7739, 4.7136) knots 0 0 0 1 2 2 2
  spline S56 degree 2 poles (-63.7739, 4.7136) (-63.8253, 4.6135) (-63.8561, 4.3771) (-63.8561, 4.1588) knots 0 0 0 1 2 2 2
  line L90 (-63.8561, 4.1588) -> (-63.8561, 3.6809)
  line L91 (-63.8561, 3.6809) -> (-62.6847, 3.6809)
  line L92 (-62.6847, 3.6809) -> (-62.6847, 4.0226)
  spline S57 degree 2 poles (-62.6847, 4.0226) (-62.6847, 4.3001) (-62.7361, 4.6186) (-62.8183, 4.7419) knots 0 0 0 1 2 2 2
  spline S58 degree 2 poles (-62.8183, 4.7419) (-62.9031, 4.8601) (-63.1137, 4.9705) (-63.2807, 4.9705) knots 0 0 0 1 2 2 2
  spline S59 degree 2 poles (-64.7218, 4.8215) (-64.8349, 4.8215) (-65.0044, 4.7445) (-65.0532, 4.6597) knots 0 0 0 1 2 2 2
  spline S60 degree 2 poles (-65.0532, 4.6597) (-65.1097, 4.5569) (-65.1354, 4.3078) (-65.1354, 4.0843) knots 0 0 0 1 2 2 2
  line L93 (-65.1354, 4.0843) -> (-65.1354, 3.6809)
  line L94 (-65.1354, 3.6809) -> (-64.2081, 3.6809)
  line L95 (-64.2081, 3.6809) -> (-64.2081, 4.1588)
  spline S61 degree 2 poles (-64.2081, 4.1588) (-64.2081, 4.3566) (-64.2492, 4.5441) (-64.3134, 4.6443) knots 0 0 0 1 2 2 2
  spline S62 degree 2 poles (-64.3134, 4.6443) (-64.375, 4.7419) (-64.5728, 4.8215) (-64.7218, 4.8215) knots 0 0 0 1 2 2 2
  spline S63 degree 2 poles (-65.1329, 8.0712) (-64.9222, 8.251) (-64.3057, 8.4514) (-63.9101, 8.4514) knots 0 0 0 1 2 2 2
  spline S64 degree 2 poles (-63.9101, 8.4514) (-63.5247, 8.4514) (-62.9005, 8.2561) (-62.6899, 8.0712) knots 0 0 0 1 2 2 2
  spline S65 degree 2 poles (-62.6899, 8.0712) (-62.4689, 7.8759) (-62.2583, 7.3596) (-62.2583, 7.0488) knots 0 0 0 1 2 2 2
  spline S66 degree 2 poles (-62.2583, 7.0488) (-62.2583, 6.7276) (-62.4766, 6.2139) (-62.6899, 6.0263) knots 0 0 0 1 2 2 2
  spline S67 degree 2 poles (-62.6899, 6.0263) (-62.9005, 5.8439) (-63.5196, 5.6487) (-63.9101, 5.6487) knots 0 0 0 1 2 2 2
  spline S68 degree 2 poles (-63.9101, 5.6487) (-64.3083, 5.6487) (-64.9145, 5.8465) (-65.1329, 6.0289) knots 0 0 0 1 2 2 2
  spline S69 degree 2 poles (-65.1329, 6.0289) (-65.3435, 6.2139) (-65.5619, 6.7302) (-65.5619, 7.0488) knots 0 0 0 1 2 2 2
  spline S70 degree 2 poles (-65.5619, 7.0488) (-65.5619, 7.3724) (-65.3358, 7.8913) (-65.1329, 8.0712) knots 0 0 0 1 2 2 2
  spline S71 degree 2 poles (-63.9101, 8.0121) (-64.2235, 8.0121) (-64.709, 7.8759) (-64.8683, 7.7526) knots 0 0 0 1 2 2 2
  spline S72 degree 2 poles (-64.8683, 7.7526) (-65.0327, 7.6268) (-65.1971, 7.2722) (-65.1971, 7.0513) knots 0 0 0 1 2 2 2
  spline S73 degree 2 poles (-65.1971, 7.0513) (-65.1971, 6.8227) (-65.0378, 6.4785) (-64.8683, 6.3474) knots 0 0 0 1 2 2 2
  spline S74 degree 2 poles (-64.8683, 6.3474) (-64.7064, 6.2216) (-64.2183, 6.088) (-63.9101, 6.088) knots 0 0 0 1 2 2 2
  spline S75 degree 2 poles (-63.9101, 6.088) (-63.2858, 6.088) (-62.6231, 6.612) (-62.6231, 7.0513) knots 0 0 0 1 2 2 2
  spline S76 degree 2 poles (-62.6231, 7.0513) (-62.6231, 7.4906) (-63.2858, 8.0121) (-63.9101, 8.0121) knots 0 0 0 1 2 2 2
  line L96 (-62.3251, 10.0184) -> (-62.3251, 8.7905)
  line L97 (-62.3251, 8.7905) -> (-62.6488, 8.7905)
  line L98 (-62.6488, 8.7905) -> (-62.6488, 9.1938)
  line L99 (-62.6488, 9.1938) -> (-65.1714, 9.1938)
  line L100 (-65.1714, 9.1938) -> (-65.1714, 8.7905)
  line L101 (-65.1714, 8.7905) -> (-65.4951, 8.7905)
  line L102 (-65.4951, 8.7905) -> (-65.4951, 10.0184)
  line L103 (-65.4951, 10.0184) -> (-65.1714, 10.0184)
  line L104 (-65.1714, 10.0184) -> (-65.1714, 9.6151)
  line L105 (-65.1714, 9.6151) -> (-62.6488, 9.6151)
  line L106 (-62.6488, 9.6151) -> (-62.6488, 10.0184)
  line L107 (-62.6488, 10.0184) -> (-62.3251, 10.0184)
  line L108 (-62.3251, 12.3766) -> (-62.3251, 10.5399)
  line L109 (-62.3251, 10.5399) -> (-65.4951, 10.5399)
  line L110 (-65.4951, 10.5399) -> (-65.4951, 10.9612)
  line L111 (-65.4951, 10.9612) -> (-62.7001, 10.9612)
  line L112 (-62.7001, 10.9612) -> (-62.7001, 12.3766)
  line L113 (-62.7001, 12.3766) -> (-62.3251, 12.3766)
  spline S77 degree 2 poles (-65.1329, 14.9506) (-64.9222, 15.1305) (-64.3057, 15.3308) (-63.9101, 15.3308) knots 0 0 0 1 2 2 2
  spline S78 degree 2 poles (-63.9101, 15.3308) (-63.5247, 15.3308) (-62.9005, 15.1356) (-62.6899, 14.9506) knots 0 0 0 1 2 2 2
  spline S79 degree 2 poles (-62.6899, 14.9506) (-62.4689, 14.7554) (-62.2583, 14.2391) (-62.2583, 13.9282) knots 0 0 0 1 2 2 2
  spline S80 degree 2 poles (-62.2583, 13.9282) (-62.2583, 13.6071) (-62.4766, 13.0933) (-62.6899, 12.9058) knots 0 0 0 1 2 2 2
  spline S81 degree 2 poles (-62.6899, 12.9058) (-62.9005, 12.7234) (-63.5196, 12.5282) (-63.9101, 12.5282) knots 0 0 0 1 2 2 2
  spline S82 degree 2 poles (-63.9101, 12.5282) (-64.3083, 12.5282) (-64.9145, 12.726) (-65.1329, 12.9084) knots 0 0 0 1 2 2 2
  spline S83 degree 2 poles (-65.1329, 12.9084) (-65.3435, 13.0933) (-65.5619, 13.6097) (-65.5619, 13.9282) knots 0 0 0 1 2 2 2
  spline S84 degree 2 poles (-65.5619, 13.9282) (-65.5619, 14.2519) (-65.3358, 14.7708) (-65.1329, 14.9506) knots 0 0 0 1 2 2 2
  spline S85 degree 2 poles (-63.9101, 14.8915) (-64.2235, 14.8915) (-64.709, 14.7554) (-64.8683, 14.6321) knots 0 0 0 1 2 2 2
  spline S86 degree 2 poles (-64.8683, 14.6321) (-65.0327, 14.5062) (-65.1971, 14.1517) (-65.1971, 13.9308) knots 0 0 0 1 2 2 2
  spline S87 degree 2 poles (-65.1971, 13.9308) (-65.1971, 13.7022) (-65.0378, 13.3579) (-64.8683, 13.2269) knots 0 0 0 1 2 2 2
  spline S88 degree 2 poles (-64.8683, 13.2269) (-64.7064, 13.101) (-64.2183, 12.9675) (-63.9101, 12.9675) knots 0 0 0 1 2 2 2
  spline S89 degree 2 poles (-63.9101, 12.9675) (-63.2858, 12.9675) (-62.6231, 13.4915) (-62.6231, 13.9308) knots 0 0 0 1 2 2 2
  spline S90 degree 2 poles (-62.6231, 13.9308) (-62.6231, 14.3701) (-63.2858, 14.8915) (-63.9101, 14.8915) knots 0 0 0 1 2 2 2
  point P0 (0, 0)
  constraints: 2 other
extrude "Wyciągnięcie proste4" cut sketch "Szkic6" against normal blind 1
sketch "Szkic8" plane through (0, 15, 0) normal (0, 1, 0) x (1, 0, 0)
  line L0 (-16.5238, -42.1509) -> (-19.5238, -42.1509)
  line L1 (-19.5238, -42.1509) -> (-19.5238, -45.1509)
  line L2 (-19.5238, -45.1509) -> (-16.5238, -45.1509)
  line L3 (-16.5238, -45.1509) -> (-16.5238, -42.1509)
  line L4 (-10.7105, -40.6509) -> (-45.2105, -40.6509) projected
  point P0 (0, 0)
  dimension "d23" = 3
  dimension "d24" = 3
  dimension "d25" = 1.5
  constraints: 8 end point, 2 parallel, 1 horizontal, 1 perpendicular
  measures "d23" distance of L2.end L1.end
  measures "d24" distance of L1.end L0.end
  measures "d25" distance between parallel lines of L4 L0
sketch "Szkic9" plane through (0, 0, 0) normal (0, -1, 0) x (1, 0, 0)
  circle A0 centre (-20.2105, -48.3969) radius 1.75
  line L0 (-4.7105, -51.3969) -> (-51.2105, -51.3969) projected
  line L1 (-4.7105, 46.6031) -> (-4.7105, -51.3969) projected
  circle A1 centre (-48.2105, -40.3969) radius 1.75
  line L2 (-51.2105, -51.3969) -> (-51.2105, -29.3969) projected
  circle A2 centre (-78.7295, -11.3969) radius 1.75
  circle A3 centre (-35.7105, -48.3969) radius 1.75
  line L3 (-51.2105, -29.3969) -> (-81.7295, -29.3969) projected
  circle A4 centre (-78.7295, 6.6031) radius 1.75
  line L4 (-81.7295, 24.6031) -> (-51.2105, 24.6031) projected
  line L5 (-81.7295, -29.3969) -> (-81.7295, 24.6031) projected
  circle A5 centre (-64.97, -26.3969) radius 1.75
  circle A6 centre (-64.97, 21.6031) radius 1.75
  circle A7 centre (-48.2105, 35.6031) radius 1.75
  line L6 (-51.2105, 46.6031) -> (-4.7105, 46.6031) projected
  circle A8 centre (-33.9605, 43.6031) radius 1.75
  circle A9 centre (-20.2105, 42.6031) radius 1.75
  circle A10 centre (-7.7105, -18.7302) radius 1.75
  circle A11 centre (-7.7105, 13.9365) radius 1.75
  point P0 (0, 0)
  dimension "d26" = 3.5
  dimension "d27" = 3
  dimension "d28" = 15.5
  dimension "d29" = 3.5
  dimension "d30" = 3
  dimension "d31" = 3.5
  dimension "d32" = 11
  dimension "d33" = 3.5
  dimension "d34" = 15.5
  dimension "d35" = 18
  dimension "d36" = 3.5
  dimension "d37" = 18
  dimension "d38" = 3
  dimension "d39" = 3
  dimension "d40" = 3.5
  dimension "d41" = 16.7595
  dimension "d42" = 3
  dimension "d43" = 3.5
  dimension "d44" = 3
  dimension "d45" = 3.5
  dimension "d46" = 11
  dimension "d47" = 3.5
  dimension "d48" = 3
  dimension "d49" = 3.5
  dimension "d50" = 4
  dimension "d51" = 3.5
  dimension "d52" = 3
  dimension "d53" = 32.6667
  dimension "d54" = 3.5
  dimension "d55" = 32.6667
  constraints: 12 centre point
  measures "d26" diameter of A0
  measures "d27" distance from line of L0 A0.centre
  measures "d28" distance from line of A0.centre L1
  measures "d29" diameter of A1
  measures "d30" distance from line of L2 A1.centre
  measures "d31" diameter of A2
  measures "d32" distance from line of L0 A1.centre
  measures "d33" diameter of A3
  measures "d34" distance from line of L2 A3.centre
  measures "d35" distance from line of L3 A2.centre
  measures "d36" diameter of A4
  measures "d37" distance from line of L4 A4.centre
  measures "d38" distance from line of L5 A4.centre
  measures "d39" distance from line of L5 A2.centre
  measures "d40" diameter of A5
  measures "d41" distance from line of A5.centre L5
  measures "d42" distance from line of L3 A5.centre
  measures "d43" diameter of A6
  measures "d44" distance from line of A6.centre L4
  measures "d45" diameter of A7
  measures "d46" distance from line of L6 A7.centre
  measures "d47" diameter of A8
  measures "d48" distance from line of L6 A8.centre
  measures "d49" diameter of A9
  measures "d50" distance from line of A9.centre L6
  measures "d51" diameter of A10
  measures "d52" distance from line of L1 A10.centre
  measures "d53" distance from line of L0 A10.centre
  measures "d54" diameter of A11
  measures "d55" distance from line of L6 A11.centre
extrude "Wyciągnięcie proste5" cut sketch "Szkic9" against normal blind 27
sketch "Szkic10" plane through (0, 0, 0) normal (0, -1, 0) x (1, 0, 0)
  line L0 (-45.2105, 18.6031) -> (-75.7295, 18.6031) projected
  line L1 (-56.1424, 18.6031) -> (-43.8424, 18.6031)
  line L2 (-43.8424, 18.6031) -> (-43.8424, -0.3969)
  line L3 (-43.8424, -0.3969) -> (-56.1424, -0.3969)
  line L4 (-56.1424, -0.3969) -> (-56.1424, 18.6031)
  point P0 (0, 0)
  dimension "d58" = 12.3
  dimension "d59" = 19
  constraints: 8 end point, 2 parallel, 1 horizontal, 1 perpendicular, 1 point on line
  measures "d58" distance of L2.end L3.end
  measures "d59" distance of L1.end L2.end
extrude "Wyciągnięcie proste6" cut sketch "Szkic10" against normal blind 2
sketch "Szkic15" plane through (-4.7105, 0, -51.3969) normal (0, 0, -1) x (-1, 0, 0)
  line L0 (0, 15) -> (46.5, 15) projected
  line L1 (0, 15) -> (5.517, 15)
  line L2 (5.517, 15) -> (13.778, 0)
  line L3 (0, 0) -> (46.5, 0) projected
  line L4 (13.778, 0) -> (0, 0)
  line L5 (0, 0) -> (0, 15) projected
  line L6 (0, 0) -> (0, 15)
  point P0 (-4.7105, 0)
  dimension "d66" = 5.517
  constraints: 8 end point, 2 point on line, 1 collinear, 1 horizontal
  measures "d66" distance of L0.start L1.end
extrude "Wyciągnięcie proste8" cut sketch "Szkic15" against normal blind 98
sketch "Szkic17" plane through (-51.2105, 0, -51.3969) normal (0, 0, -1) x (-1, 0, 0)
  line L0 (-32.75, 0.0509) -> (-32.722, 0) projected
  line L1 (-32.722, 0) -> (-29.722, 0)
  line L2 (-29.25, 0) -> (-32.722, 0) projected
  line L3 (-40.983, 15) -> (0, 15) projected
  line L4 (-40.983, 15) -> (-37.983, 15)
  line L5 (-37.983, 15) -> (-29.722, 0)
  line L6 (-32.75, 0.0509) -> (-40.983, 15)
  point P0 (-51.2105, 0)
  dimension "d77" = 3
  dimension "d78" = 3
  constraints: 8 end point, 2 point on line
  measures "d77" distance of L0.end L1.end
  measures "d78" distance of L3.start L4.end
extrude "Wyciągnięcie proste10" cut sketch "Szkic17" against normal blind 98
sketch "Szkic18" plane through (0, 0, 0) normal (0, -1, 0) x (1, 0, 0)
  arc A0 (-21.4886, -47.2014) -> (-21.4886, -49.5924) centre (-20.2105, -48.3969) ccw projected
  circle A1 centre (-20.2105, -48.3969) radius 1.75
  circle A2 centre (-20.2105, 42.6031) radius 1.75 projected
  circle A3 centre (-20.2105, 42.6031) radius 1.75
  point P0 (0, 0)
  constraints: 2 centre point, 2 coincident
extrude "Wyciągnięcie proste11" add sketch "Szkic18" against normal blind 15
sketch "Szkic19" plane through (0, 0, 0) normal (0, -1, 0) x (1, 0, 0)
  point P0 (0, 0)
chamfer "Faza1" distance 0.8 angle 45 8 edges at (-49.9605, 0, -40.3969) (-37.4605, 0, -48.3969) (-66.72, 0, -26.3969) (-80.4795, 0, -11.3969) (-80.4795, 0, 6.6031) (-66.72, 0, 21.6031) (-49.9605, 0, 35.6031) (-35.7105, 0, 43.6031)
sketch "Szkic20" plane through (0, 0, 0) normal (0, -1, 0) x (1, 0, 0)
  line L0 (-56.1424, -0.3969) -> (-56.1424, 18.6031) projected
  line L1 (-56.1424, 18.6031) -> (-43.8424, 18.6031) projected
  line L2 (-56.1424, -0.3969) -> (-43.8424, -0.3969)
  line L3 (-43.8424, -0.3969) -> (-43.8424, 18.6031)
  line L4 (-43.8424, 18.6031) -> (-56.1424, 18.6031)
  line L5 (-56.1424, 18.6031) -> (-56.1424, -0.3969)
  point P0 (0, 0)
  constraints: 8 end point, 2 parallel, 1 horizontal, 1 perpendicular
extrude "Wyciągnięcie proste12" add sketch "Szkic20" against normal blind 2
sketch "Szkic21" plane through (0, 0, 0) normal (0, -1, 0) x (1, 0, 0)
  line L0 (-64.2127, -5.8882) -> (-54.2127, -5.8882)
  line L1 (-54.2127, -5.8882) -> (-54.2127, -20.8882)
  line L2 (-54.2127, -20.8882) -> (-64.2127, -20.8882)
  line L3 (-64.2127, -20.8882) -> (-64.2127, -5.8882)
  point P0 (0, 0)
  dimension "d88" = 10
  dimension "d89" = 15
  constraints: 8 end point, 2 parallel, 1 horizontal, 1 perpendicular
  measures "d88" distance of L1.end L2.end
  measures "d89" distance of L0.end L1.end
extrude "Wyciągnięcie proste13" cut sketch "Szkic21" against normal blind 2
sketch "Szkic22" plane through (0, 0, 0) normal (0, -1, 0) x (1, 0, 0)
  circle A0 centre (-35.7105, -48.3969) radius 1.75 projected
  circle A1 centre (-35.7105, -48.3969) radius 1.75
  circle A2 centre (-35.7105, -48.3969) radius 2.55
  point P0 (0, 0)
  constraints: 2 centre point, 2 coincident
extrude "Wyciągnięcie proste14" add sketch "Szkic22" against normal blind 15 contours A0
extrude "Wyciągnięcie proste15" add sketch "Szkic8" along normal blind 15
sketch "Szkic23" plane through (0, 0, 0) normal (0, -1, 0) x (1, 0, 0)
  circle A0 centre (-35.7105, -48.3969) radius 2.55 projected
  circle A1 centre (-35.7105, -48.3969) radius 2.55
  point P0 (0, 0)
  constraints: 1 centre point, 1 coincident
extrude "Wyciągnięcie proste16" add sketch "Szkic23" against normal blind 15
sketch "Szkic24" plane through (0, 0, 0) normal (0, -1, 0) x (1, 0, 0)
  circle A0 centre (-33.9415, -48.3969) radius 1.75
  line L0 (-51.2105, -51.3969) -> (-51.2105, -29.3969) projected
  line L1 (-21.4886, -51.3969) -> (-51.2105, -51.3969) projected
  point P0 (0, 0)
  dimension "d98" = 3.5
  dimension "d99" = 17.269
  dimension "d100" = 3
  constraints: 1 centre point
  measures "d98" diameter of A0
  measures "d99" distance from line of L0 A0.centre
  measures "d100" distance from line of L1 A0.centre
extrude "Wyciągnięcie proste17" cut sketch "Szkic24" against normal blind 15
chamfer "Faza2" distance 0.8 angle 45 1 edges at (-35.6915, 0, -48.3969)
sketch "Szkic25" plane through (0, 30, 0) normal (0, 1, 0) x (1, 0, 0)
  line L0 (-16.5238, -42.1509) -> (-16.5238, -45.1509) projected
  line L1 (-19.5238, -45.1509) -> (-19.5238, -42.1509) projected
  line L2 (-16.5238, -42.1509) -> (-19.5238, -42.1509)
  line L3 (-19.5238, -42.1509) -> (-19.5238, -45.1509)
  line L4 (-19.5238, -45.1509) -> (-16.5238, -45.1509)
  line L5 (-16.5238, -45.1509) -> (-16.5238, -42.1509)
  point P0 (0, 0)
  constraints: 8 end point, 2 parallel, 1 horizontal, 1 perpendicular
extrude "Wyciągnięcie proste18" cut sketch "Szkic25" against normal blind 15
